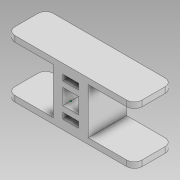
# Autodesk Inventor part: fuselage_tail_interface_back
Saved by Autodesk Inventor 2021 (Build 250183000, 183)
## iProperties
Created: 2020-12-06
Part Number: fuselage_tail_interface_back
Material: Generic
Document SubType Name: Modeling
Designer: victo
Density: 1 g/cm^3
Appearance: Default
Mass: 1.7836 g
Surface Area: 21.6474 cm^2
Volume: 1.7836 cm^3
Author: victo
Autodesk Inventor part; units mm, degrees
ref_plane "YZ Plane" through (0, 0, 0) normal (1, 0, 0) x (0, 1, 0)
ref_plane "XZ Plane" through (0, 0, 0) normal (0, 1, 0) x (-1, 0, 0)
ref_plane "XY Plane" through (0, 0, 0) normal (0, 0, 1) x (1, 0, 0)
sketch "Sketch1" plane through (0, 0, 0) normal (0, 0, 1) x (1, 0, 0)
  line L0 (-4.55, 7.5) -> (4.55, 7.5)
  line L1 (4.55, 7.5) -> (4.55, -7.5)
  line L2 (4.55, -7.5) -> (-4.55, -7.5)
  line L3 (-4.55, -7.5) -> (-4.55, 7.5)
  line L4 (-4.55, 7.5) -> (4.55, -7.5) construction
  line L5 (4.55, 7.5) -> (-4.55, -7.5) construction
  line L6 (-2.05, -2.05) -> (2.05, -2.05)
  line L7 (2.05, -2.05) -> (2.05, 2.05)
  line L8 (2.05, 2.05) -> (-2.05, 2.05)
  line L9 (-2.05, 2.05) -> (-2.05, -2.05)
  line L10 (-2.05, -2.05) -> (2.05, 2.05) construction
  line L11 (2.05, -2.05) -> (-2.05, 2.05) construction
  line L12 (-4.55, 7.5) -> (-16.55, 7.5)
  line L13 (-16.55, 7.5) -> (-16.55, 6)
  line L14 (-16.55, 6) -> (-4.55, 6)
  line L15 (-4.55, 6) -> (-4.55, 7.5)
  line L16 (-4.55, -7.5) -> (-16.55, -7.5)
  line L17 (-16.55, -7.5) -> (-16.55, -6)
  line L18 (-16.55, -6) -> (-4.55, -6)
  line L19 (-4.55, -6) -> (-4.55, -7.5)
  line L20 (4.55, 7.5) -> (16.55, 7.5)
  line L21 (16.55, 7.5) -> (16.55, 6)
  line L22 (16.55, 6) -> (4.55, 6)
  line L23 (4.55, 6) -> (4.55, 7.5)
  line L24 (4.55, -7.5) -> (16.55, -7.5)
  line L25 (16.55, -7.5) -> (16.55, -6)
  line L26 (16.55, -6) -> (4.55, -6)
  line L27 (4.55, -6) -> (4.55, -7.5)
  point P0 (0, 0)
  point P1 (-4.55, 6)
  point P2 (-4.55, -6)
  point P3 (4.55, 6)
  dimension "d0" = 15
  dimension "d1" = 9.1
  dimension "d2" = 4.1
  dimension "d3" = 4.1
  dimension "d4" = 12
  dimension "d5" = 1.5
  dimension "d8" = 1.5
  dimension "d9" = 12
  dimension "d10" = 12
  dimension "d11" = 1.5
  dimension "d12" = 12
  constraints: 56 end point, 12 parallel, 6 horizontal, 6 perpendicular, 4 midpoint, 1 point on line
  measures "d0" distance of L0.end L1.end
  measures "d1" distance of L0.start L0.end
  measures "d2" distance of L7.end L8.end
  measures "d3" distance of L6.end L7.end
  measures "d4" distance of L21.end L22.end
  measures "d5" distance of L20.end L21.end
  measures "d8" distance of L16.end L17.end
  measures "d9" distance of L0.start L12.end
  measures "d10" distance of L17.end L18.end
  measures "d11" distance of L24.end L25.end
  measures "d12" distance of L25.end L26.end
extrude "Extrusion1" add sketch "Sketch1" along normal blind 10
sketch "Sketch2" plane through (0, 0, 10) normal (0, 0, 1) x (1, 0, 0)
  point P0 (0, 0)
fillet "Fillet1" radius 2 8 edges at (-16.55, 6.75, 10) (-16.55, -6.75, 10) (16.55, -6.75, 10) (16.55, 6.75, 10) (16.55, 6.75, 0) (-16.55, 6.75, 0) (-16.55, -6.75, 0) (16.55, -6.75, 0)
sketch "Sketch3" plane through (0, 0, 0) normal (0, 0, -1) x (-1, 0, 0)
  line L0 (-2.05, 5.05) -> (2.05, 5.05)
  line L1 (2.05, 5.05) -> (2.05, 3.55)
  line L2 (2.05, 3.55) -> (-2.05, 3.55)
  line L3 (-2.05, 3.55) -> (-2.05, 5.05)
  line L4 (-2.05, -3.55) -> (2.05, -3.55)
  line L5 (2.05, -3.55) -> (2.05, -5.05)
  line L6 (2.05, -5.05) -> (-2.05, -5.05)
  line L7 (-2.05, -5.05) -> (-2.05, -3.55)
  line L8 (-2.05, 2.05) -> (-2.05, -2.05) projected
  line L9 (2.05, -2.05) -> (2.05, 2.05) projected
  line L10 (2.05, 2.05) -> (-2.05, 2.05) projected
  line L11 (-2.05, -2.05) -> (2.05, -2.05) projected
  point P0 (0, 0)
  dimension "d16" = 1.5
  dimension "d17" = 1.5
  dimension "d18" = 1.5
  dimension "d19" = 1.5
  constraints: 16 end point, 4 parallel, 3 collinear, 2 horizontal, 2 perpendicular, 1 point on line
  measures "d16" distance between parallel lines of L10 L2
  measures "d17" distance between parallel lines of L11 L4
  measures "d18" distance between parallel lines of L2 L0
  measures "d19" distance of L4.end L5.end
extrude "Extrusion2" cut sketch "Sketch3" against normal blind 10 contours L0 L1 L2 L3 | L4 L5 L6 L7
body "Solid1"
